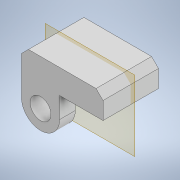
# Autodesk Inventor part: 2번부품
Saved by Autodesk Inventor 2022 (Build 260153000, 153)
## iProperties
Created: 2021-09-11
Part Number: 2번부품
Material: 일반
Document SubType Name: Modeling
Designer: 서울공업고등학교
Density: 1 g/cm^3
Appearance: 기본값
Author: 서울공업고등학교
Autodesk Inventor part; units mm, degrees
ref_plane "YZ Plane" through (0, 0, 0) normal (1, 0, 0) x (0, 1, 0)
ref_plane "XZ Plane" through (0, 0, 0) normal (0, 1, 0) x (-1, 0, 0)
ref_plane "XY Plane" through (0, 0, 0) normal (0, 0, 1) x (1, 0, 0)
sketch "스케치1" plane through (0, 0, 0) normal (0, 0, 1) x (1, 0, 0)
  line L0 (0, 0) -> (23.5, 0)
  line L1 (23.5, 0) -> (23.5, -7)
  line L2 (23.5, -7) -> (11, -7)
  line L3 (0, -7) -> (0, 0)
  circle A0 centre (5.5, -13) radius 3
  arc A1 (0, -13) -> (11, -13) centre (5.5, -13) ccw
  line L4 (11, -13) -> (11, -7)
  line L5 (0, -13) -> (0, -7)
  dimension "d0" = 23.5
  dimension "d1" = 7
  dimension "d2" = 6
  dimension "d3" = 6
  dimension "d4" = 5.5
  dimension "d5" = 11
  dimension "d6" = 23.5
  constraints: 12 end point, 2 centre point, 2 parallel, 2 perpendicular, 2 point on circle, 2 tangent, 1 coincident, 1 horizontal
  measures "d0" distance of L1.end L3.start
  measures "d1" distance of L0.end L1.end
  measures "d2" diameter of A0
  measures "d3" distance from line of L2 A0.centre
  measures "d4" horizontal distance of L0.start A0.centre
  measures "d5" diameter of A1
  measures "d6" distance between parallel lines of L1 L3
extrude "돌출1" add sketch "스케치1" along normal mid plane 16
ref_plane "작업 평면1" through (0, 0, 0) normal (0, 0, 1) x (1, 0, 0)
sketch "스케치2" plane through (0, 0, 0) normal (0, 0, 1) x (1, 0, 0)
  line L0 (-2.9119, -7) -> (15.7404, -7)
  line L1 (15.7404, -7) -> (15.7404, -20.77)
  line L2 (15.7404, -20.77) -> (-2.9119, -20.77)
  line L3 (-2.9119, -20.77) -> (-2.9119, -7)
  line L4 (0, 0) -> (23.5, 0) projected
  dimension "d9" = 7
  constraints: 8 end point, 2 parallel, 1 horizontal, 1 perpendicular
  measures "d9" distance between parallel lines of L0 L4
extrude "돌출2" cut sketch "스케치2" along normal mid plane 7
chamfer "모따기1" distance 2 angle 45 2 edges at (23.5, 0, 0) (0, 0, 0)
